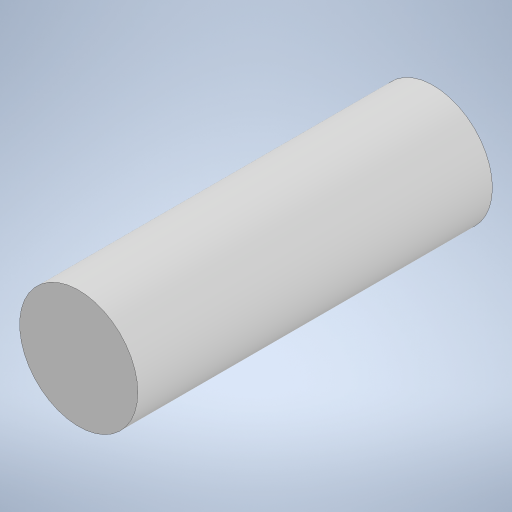
# Autodesk Inventor part: bolt
Saved by Autodesk Inventor 2024 (Build 280153000, 153)
## iProperties
Created: 2024-08-23
Part Number: bolt
Material: Generic
Document SubType Name: Modeling
Designer: domko
Density: 1 g/cm^3
Appearance: Default
Author: domko
Autodesk Inventor part; units mm, degrees
ref_plane "YZ Plane" through (0, 0, 0) normal (1, 0, 0) x (0, 1, 0)
ref_plane "XZ Plane" through (0, 0, 0) normal (0, 1, 0) x (-1, 0, 0)
ref_plane "XY Plane" through (0, 0, 0) normal (0, 0, 1) x (1, 0, 0)
sketch "Sketch1" plane through (0, 0, 0) normal (0, 0, 1) x (1, 0, 0)
  circle A0 centre (0, 0) radius 5
  dimension "d0" = 10
  constraints: 1 centre point, 1 coincident
  measures "d0" diameter of A0
extrude "Extrusion1" add sketch "Sketch1" along normal blind 30
body "Solid1"
